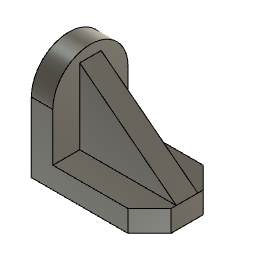
a1 (Autodesk Fusion 360 design; units mm, degrees)
Autodesk Fusion 360 part; units mm, degrees
sketch "Sketch1" plane through (0, 0, 0) normal (0, 0, 1) x (1, 0, 0)
  line L0 (0, 0) -> (66, 0) construction
  line L1 (66, 0) -> (66, -42) construction
  line L2 (66, -42) -> (0, -42) construction
  line L3 (0, -42) -> (0, 0)
  line L4 (66, 0) -> (54, 0) construction
  line L5 (54, 0) -> (54, -12) construction
  line L6 (54, -12) -> (66, -12) construction
  line L7 (66, -12) -> (66, 0) construction
  line L8 (66, -42) -> (54, -42) construction
  line L9 (54, -42) -> (54, -30) construction
  line L10 (54, -30) -> (66, -30) construction
  line L11 (66, -30) -> (66, -42) construction
  line L12 (54, 0) -> (66, -12)
  line L13 (66, -30) -> (54, -42)
  line L14 (0, -42) -> (54, -42)
  line L15 (0, 0) -> (54, 0)
  line L16 (66, -12) -> (66, -30)
  line L17 (0, 0) -> (12, 0)
  line L18 (12, 0) -> (12, -42)
  line L19 (12, -42) -> (0, -42)
  line L20 (0, -42) -> (0, 0)
  line L21 (66, -21) -> (12, -21)
  line L22 (12, -21) -> (12, -15)
  line L23 (12, -21) -> (12, -27)
  line L24 (12, -27) -> (66, -27)
  line L25 (12, -15) -> (66, -15)
  dimension "d1" = 66
  dimension "d2" = 42
  dimension "d3" = 12
  dimension "d4" = 12
  dimension "d5" = 12
  dimension "d6" = 12
  dimension "d7" = 42
  dimension "d8" = 12
  dimension "d9" = 6
  dimension "d10" = 6
  constraint horizontal L0
  constraint vertical L1
  constraint horizontal L2
  constraint vertical L3
  constraint coincident L0.start L3.end
  constraint horizontal L4
  constraint vertical L5
  constraint horizontal L6
  constraint vertical L7
  constraint horizontal L8
  constraint vertical L9
  constraint horizontal L10
  constraint vertical L11
  constraint horizontal L17
  constraint vertical L18
  constraint horizontal L19
  constraint vertical L20
  constraint midpoint L16 L21.start
  constraint midpoint L18 L21.end
  constraint perpendicular L21 L22
  constraint perpendicular L21 L23
  constraint coincident L1 L24.end
  constraint coincident L16 L25.end
  measures "d1" distance of L0.start L0.end
  measures "d2" distance of L0.start L2.end
  measures "d3" distance of L0.end L6.end
  measures "d4" distance of L0.end L4.end
  measures "d5" distance of L1.end L10.end
  measures "d6" distance of L1.end L8.end
  measures "d7" distance of L0.start L2.end
  measures "d8" distance of L0.start L17.end
  measures "d9" distance of L21.end L22.end
  measures "d10" distance of L21.end L23.end
extrude "Extrude1" add sketch "Sketch1" along normal blind 60 contours L3 L14 L15 L17 L18 L19 L20 L22 L23 makes body 1
extrude "Extrude2" add sketch "Sketch1" along normal blind 12 contours L13 L14 L16 L18 L24 | L12 L15 L16 L18 L25 | L16 L18 L21 L23 L24 | L16 L18 L21 L22 L25 bodies 1
sketch "Sketch2" plane through (0, 0, 0) normal (-1, 0, 0) x (0, -1, 0)
  line L0 (0, 0) -> (42, 0)
  line L1 (42, 0) -> (42, 60)
  line L2 (42, 60) -> (0, 60)
  line L3 (0, 60) -> (0, 0)
  line L4 (0, 60) -> (42, 60)
  line L5 (42, 60) -> (42, 0)
  line L6 (42, 0) -> (0, 0)
  line L7 (0, 0) -> (0, 60)
  circle A0 centre (21, 39) radius 21
  dimension "d15" = 42
  constraint horizontal L4
  constraint vertical L5
  constraint horizontal L6
  constraint vertical L7
  constraint coincident L0.end L1.start
  constraint coincident L2.end L3.start
  constraint tangent L4 A0
  measures "d15" diameter of A0
extrude "Extrude3" cut sketch "Sketch2" against normal blind 15 contours L2 L3 L4 L7 A0 | L1 L2 L4 L5 A0 bodies 1
extrude "Extrude4" add sketch "Sketch1" along normal blind 54 separate body contours L16 L18 L21 L23 L24 | L16 L18 L21 L22 L25 makes body 2
sketch "Sketch3" plane through (0, -15, 0) normal (0, 1, 0) x (-1, 0, 0)
  line L0 (-66, 0) -> (-12, 0)
  line L1 (-12, 0) -> (-12, 54)
  line L2 (-12, 54) -> (-66, 54)
  line L3 (-66, 54) -> (-66, 0)
  line L4 (-66, 11.9878) -> (-12, 54)
  constraint coincident L3 L4.start
  constraint coincident L1.end L2.start
extrude "Extrude5" cut sketch "Sketch3" against normal blind 25 contours L2 L3 L4 bodies 1 2
combine "Combine1" operation add target body 1 tool bodies 2
